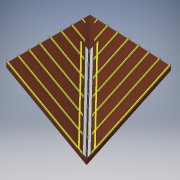
# Autodesk Inventor part: DeszkazatEsSzarufa
Saved by Autodesk Inventor 2019 (Build 230136000, 136)
## iProperties
Created: 2022-04-03
Part Number: DeszkazatEsSzarufa
Material: Generic
Document SubType Name: Modeling
Designer: laca
Density: 1 g/cm^3
Appearance: Default
Author: laca
Autodesk Inventor part; units mm, degrees
ref_plane "YZ Plane" through (0, 0, 0) normal (1, 0, 0) x (0, 1, 0)
ref_plane "XZ Plane" through (0, 0, 0) normal (0, 1, 0) x (-1, 0, 0)
ref_plane "XY Plane" through (0, 0, 0) normal (0, 0, 1) x (1, 0, 0)
sketch "Sketch1" plane through (0, 0, 0) normal (0, 0, 1) x (1, 0, 0)
  line L0 (0, 0) -> (-5247.7182, 2908.8577)
  line L1 (0, 0) -> (-5580.1481, 0)
  line L2 (0, 0) -> (-104.9544, 58.1772)
  line L3 (-104.9544, 58.1772) -> (-117.0746, 36.3117)
  line L4 (-117.0746, 36.3117) -> (-12.1202, -21.8655)
  line L5 (-12.1202, -21.8655) -> (0, 0)
  line L6 (-113.7006, 63.0253) -> (-218.6549, 121.2024)
  line L7 (-218.6549, 121.2024) -> (-230.7752, 99.3369)
  line L8 (-230.7752, 99.3369) -> (-125.8208, 41.1598)
  line L9 (-125.8208, 41.1598) -> (-113.7006, 63.0253)
  line L10 (-227.4011, 126.0505) -> (-332.3555, 184.2277)
  line L11 (-332.3555, 184.2277) -> (-344.4757, 162.3622)
  line L12 (-344.4757, 162.3622) -> (-239.5214, 104.185)
  line L13 (-239.5214, 104.185) -> (-227.4011, 126.0505)
  line L14 (-341.1017, 189.0758) -> (-446.0561, 247.2529)
  line L15 (-446.0561, 247.2529) -> (-458.1763, 225.3874)
  line L16 (-458.1763, 225.3874) -> (-353.2219, 167.2103)
  line L17 (-353.2219, 167.2103) -> (-341.1017, 189.0758)
  line L18 (-454.8022, 252.101) -> (-559.7566, 310.2782)
  line L19 (-559.7566, 310.2782) -> (-571.8769, 288.4127)
  line L20 (-571.8769, 288.4127) -> (-466.9225, 230.2355)
  line L21 (-466.9225, 230.2355) -> (-454.8022, 252.101)
  line L22 (-568.5028, 315.1263) -> (-673.4572, 373.3034)
  line L23 (-673.4572, 373.3034) -> (-685.5774, 351.4379)
  line L24 (-685.5774, 351.4379) -> (-580.6231, 293.2608)
  line L25 (-580.6231, 293.2608) -> (-568.5028, 315.1263)
  line L26 (-682.2034, 378.1515) -> (-787.1577, 436.3287)
  line L27 (-787.1577, 436.3287) -> (-799.278, 414.4632)
  line L28 (-799.278, 414.4632) -> (-694.3236, 356.286)
  line L29 (-694.3236, 356.286) -> (-682.2034, 378.1515)
  line L30 (-795.9039, 441.1768) -> (-900.8583, 499.3539)
  line L31 (-900.8583, 499.3539) -> (-912.9785, 477.4884)
  line L32 (-912.9785, 477.4884) -> (-808.0242, 419.3113)
  line L33 (-808.0242, 419.3113) -> (-795.9039, 441.1768)
  line L34 (-909.6045, 504.202) -> (-1014.5589, 562.3792)
  line L35 (-1014.5589, 562.3792) -> (-1026.6791, 540.5137)
  line L36 (-1026.6791, 540.5137) -> (-921.7247, 482.3365)
  line L37 (-921.7247, 482.3365) -> (-909.6045, 504.202)
  line L38 (-1023.3051, 567.2273) -> (-1128.2594, 625.4044)
  line L39 (-1128.2594, 625.4044) -> (-1140.3797, 603.5389)
  line L40 (-1140.3797, 603.5389) -> (-1035.4253, 545.3618)
  line L41 (-1035.4253, 545.3618) -> (-1023.3051, 567.2273)
  line L42 (-1137.0056, 630.2525) -> (-1241.96, 688.4297)
  line L43 (-1241.96, 688.4297) -> (-1254.0802, 666.5642)
  line L44 (-1254.0802, 666.5642) -> (-1149.1259, 608.387)
  line L45 (-1149.1259, 608.387) -> (-1137.0056, 630.2525)
  line L46 (-1250.7062, 693.2778) -> (-1355.6605, 751.4549)
  line L47 (-1355.6605, 751.4549) -> (-1367.7808, 729.5894)
  line L48 (-1367.7808, 729.5894) -> (-1262.8264, 671.4123)
  line L49 (-1262.8264, 671.4123) -> (-1250.7062, 693.2778)
  line L50 (-1364.4067, 756.303) -> (-1469.3611, 814.4802)
  line L51 (-1469.3611, 814.4802) -> (-1481.4813, 792.6147)
  line L52 (-1481.4813, 792.6147) -> (-1376.527, 734.4375)
  line L53 (-1376.527, 734.4375) -> (-1364.4067, 756.303)
  line L54 (-1478.1073, 819.3283) -> (-1583.0617, 877.5054)
  line L55 (-1583.0617, 877.5054) -> (-1595.1819, 855.6399)
  line L56 (-1595.1819, 855.6399) -> (-1490.2275, 797.4628)
  line L57 (-1490.2275, 797.4628) -> (-1478.1073, 819.3283)
  line L58 (-1591.8079, 882.3535) -> (-1696.7622, 940.5307)
  line L59 (-1696.7622, 940.5307) -> (-1708.8825, 918.6652)
  line L60 (-1708.8825, 918.6652) -> (-1603.9281, 860.488)
  line L61 (-1603.9281, 860.488) -> (-1591.8079, 882.3535)
  line L62 (-1705.5084, 945.3788) -> (-1810.4628, 1003.5559)
  line L63 (-1810.4628, 1003.5559) -> (-1822.583, 981.6904)
  line L64 (-1822.583, 981.6904) -> (-1717.6287, 923.5133)
  line L65 (-1717.6287, 923.5133) -> (-1705.5084, 945.3788)
  line L66 (-1819.209, 1008.404) -> (-1924.1634, 1066.5812)
  line L67 (-1924.1634, 1066.5812) -> (-1936.2836, 1044.7157)
  line L68 (-1936.2836, 1044.7157) -> (-1831.3292, 986.5385)
  line L69 (-1831.3292, 986.5385) -> (-1819.209, 1008.404)
  line L70 (-1932.9096, 1071.4293) -> (-2037.8639, 1129.6064)
  line L71 (-2037.8639, 1129.6064) -> (-2049.9842, 1107.7409)
  line L72 (-2049.9842, 1107.7409) -> (-1945.0298, 1049.5638)
  line L73 (-1945.0298, 1049.5638) -> (-1932.9096, 1071.4293)
  line L74 (-2046.6101, 1134.4545) -> (-2151.5645, 1192.6317)
  line L75 (-2151.5645, 1192.6317) -> (-2163.6847, 1170.7662)
  line L76 (-2163.6847, 1170.7662) -> (-2058.7304, 1112.589)
  line L77 (-2058.7304, 1112.589) -> (-2046.6101, 1134.4545)
  line L78 (-2160.3107, 1197.4798) -> (-2265.265, 1255.6569)
  line L79 (-2265.265, 1255.6569) -> (-2277.3853, 1233.7914)
  line L80 (-2277.3853, 1233.7914) -> (-2172.4309, 1175.6143)
  line L81 (-2172.4309, 1175.6143) -> (-2160.3107, 1197.4798)
  line L82 (-2274.0112, 1260.505) -> (-2378.9656, 1318.6822)
  line L83 (-2378.9656, 1318.6822) -> (-2391.0858, 1296.8167)
  line L84 (-2391.0858, 1296.8167) -> (-2286.1315, 1238.6395)
  line L85 (-2286.1315, 1238.6395) -> (-2274.0112, 1260.505)
  line L86 (-2387.7118, 1323.5303) -> (-2492.6662, 1381.7074)
  line L87 (-2492.6662, 1381.7074) -> (-2504.7864, 1359.8419)
  line L88 (-2504.7864, 1359.8419) -> (-2399.832, 1301.6648)
  line L89 (-2399.832, 1301.6648) -> (-2387.7118, 1323.5303)
  line L90 (-2501.4124, 1386.5555) -> (-2606.3667, 1444.7327)
  line L91 (-2606.3667, 1444.7327) -> (-2618.487, 1422.8672)
  line L92 (-2618.487, 1422.8672) -> (-2513.5326, 1364.69)
  line L93 (-2513.5326, 1364.69) -> (-2501.4124, 1386.5555)
  line L94 (-2615.1129, 1449.5808) -> (-2720.0673, 1507.7579)
  line L95 (-2720.0673, 1507.7579) -> (-2732.1875, 1485.8924)
  line L96 (-2732.1875, 1485.8924) -> (-2627.2332, 1427.7153)
  line L97 (-2627.2332, 1427.7153) -> (-2615.1129, 1449.5808)
  line L98 (-2728.8135, 1512.606) -> (-2833.7679, 1570.7832)
  line L99 (-2833.7679, 1570.7832) -> (-2845.8881, 1548.9177)
  line L100 (-2845.8881, 1548.9177) -> (-2740.9337, 1490.7405)
  line L101 (-2740.9337, 1490.7405) -> (-2728.8135, 1512.606)
  line L102 (-2842.514, 1575.6313) -> (-2947.4684, 1633.8084)
  line L103 (-2947.4684, 1633.8084) -> (-2959.5887, 1611.9429)
  line L104 (-2959.5887, 1611.9429) -> (-2854.6343, 1553.7658)
  line L105 (-2854.6343, 1553.7658) -> (-2842.514, 1575.6313)
  line L106 (-2956.2146, 1638.6565) -> (-3061.169, 1696.8337)
  line L107 (-3061.169, 1696.8337) -> (-3073.2892, 1674.9682)
  line L108 (-3073.2892, 1674.9682) -> (-2968.3349, 1616.791)
  line L109 (-2968.3349, 1616.791) -> (-2956.2146, 1638.6565)
  line L110 (-3069.9152, 1701.6818) -> (-3174.8695, 1759.8589)
  line L111 (-3174.8695, 1759.8589) -> (-3186.9898, 1737.9934)
  line L112 (-3186.9898, 1737.9934) -> (-3082.0354, 1679.8163)
  line L113 (-3082.0354, 1679.8163) -> (-3069.9152, 1701.6818)
  line L114 (-3183.6157, 1764.707) -> (-3288.5701, 1822.8842)
  line L115 (-3288.5701, 1822.8842) -> (-3300.6903, 1801.0187)
  line L116 (-3300.6903, 1801.0187) -> (-3195.736, 1742.8415)
  line L117 (-3195.736, 1742.8415) -> (-3183.6157, 1764.707)
  line L118 (-3297.3163, 1827.7323) -> (-3402.2707, 1885.9094)
  line L119 (-3402.2707, 1885.9094) -> (-3414.3909, 1864.0439)
  line L120 (-3414.3909, 1864.0439) -> (-3309.4365, 1805.8668)
  line L121 (-3309.4365, 1805.8668) -> (-3297.3163, 1827.7323)
  line L122 (-3411.0169, 1890.7575) -> (-3515.9712, 1948.9347)
  line L123 (-3515.9712, 1948.9347) -> (-3528.0915, 1927.0692)
  line L124 (-3528.0915, 1927.0692) -> (-3423.1371, 1868.892)
  line L125 (-3423.1371, 1868.892) -> (-3411.0169, 1890.7575)
  line L126 (-3524.7174, 1953.7828) -> (-3629.6718, 2011.9599)
  line L127 (-3629.6718, 2011.9599) -> (-3641.792, 1990.0944)
  line L128 (-3641.792, 1990.0944) -> (-3536.8377, 1931.9173)
  line L129 (-3536.8377, 1931.9173) -> (-3524.7174, 1953.7828)
  line L130 (-3638.418, 2016.808) -> (-3743.3723, 2074.9852)
  line L131 (-3743.3723, 2074.9852) -> (-3755.4926, 2053.1197)
  line L132 (-3755.4926, 2053.1197) -> (-3650.5382, 1994.9425)
  line L133 (-3650.5382, 1994.9425) -> (-3638.418, 2016.808)
  line L134 (-3752.1185, 2079.8333) -> (-3857.0729, 2138.0104)
  line L135 (-3857.0729, 2138.0104) -> (-3869.1931, 2116.1449)
  line L136 (-3869.1931, 2116.1449) -> (-3764.2388, 2057.9678)
  line L137 (-3764.2388, 2057.9678) -> (-3752.1185, 2079.8333)
  line L138 (-3865.8191, 2142.8585) -> (-3970.7735, 2201.0357)
  line L139 (-3970.7735, 2201.0357) -> (-3982.8937, 2179.1702)
  line L140 (-3982.8937, 2179.1702) -> (-3877.9393, 2120.993)
  line L141 (-3877.9393, 2120.993) -> (-3865.8191, 2142.8585)
  line L142 (-3979.5197, 2205.8838) -> (-4084.474, 2264.0609)
  line L143 (-4084.474, 2264.0609) -> (-4096.5943, 2242.1954)
  line L144 (-4096.5943, 2242.1954) -> (-3991.6399, 2184.0183)
  line L145 (-3991.6399, 2184.0183) -> (-3979.5197, 2205.8838)
  line L146 (-4093.2202, 2268.909) -> (-4198.1746, 2327.0862)
  line L147 (-4198.1746, 2327.0862) -> (-4210.2948, 2305.2207)
  line L148 (-4210.2948, 2305.2207) -> (-4105.3405, 2247.0435)
  line L149 (-4105.3405, 2247.0435) -> (-4093.2202, 2268.909)
  line L150 (-4206.9208, 2331.9343) -> (-4311.8752, 2390.1114)
  line L151 (-4311.8752, 2390.1114) -> (-4323.9954, 2368.2459)
  line L152 (-4323.9954, 2368.2459) -> (-4219.041, 2310.0688)
  line L153 (-4219.041, 2310.0688) -> (-4206.9208, 2331.9343)
  line L154 (-4320.6214, 2394.9595) -> (-4425.5757, 2453.1367)
  line L155 (-4425.5757, 2453.1367) -> (-4437.696, 2431.2712)
  line L156 (-4437.696, 2431.2712) -> (-4332.7416, 2373.094)
  line L157 (-4332.7416, 2373.094) -> (-4320.6214, 2394.9595)
  line L158 (-4434.3219, 2457.9848) -> (-4539.2763, 2516.1619)
  line L159 (-4539.2763, 2516.1619) -> (-4551.3965, 2494.2964)
  line L160 (-4551.3965, 2494.2964) -> (-4446.4422, 2436.1193)
  line L161 (-4446.4422, 2436.1193) -> (-4434.3219, 2457.9848)
  line L162 (-4548.0225, 2521.01) -> (-4652.9768, 2579.1872)
  line L163 (-4652.9768, 2579.1872) -> (-4665.0971, 2557.3217)
  line L164 (-4665.0971, 2557.3217) -> (-4560.1427, 2499.1445)
  line L165 (-4560.1427, 2499.1445) -> (-4548.0225, 2521.01)
  line L166 (-4661.723, 2584.0353) -> (-4766.6774, 2642.2124)
  line L167 (-4766.6774, 2642.2124) -> (-4778.7976, 2620.3469)
  line L168 (-4778.7976, 2620.3469) -> (-4673.8433, 2562.1698)
  line L169 (-4673.8433, 2562.1698) -> (-4661.723, 2584.0353)
  line L170 (-4775.4236, 2647.0605) -> (-4880.378, 2705.2377)
  line L171 (-4880.378, 2705.2377) -> (-4892.4982, 2683.3722)
  line L172 (-4892.4982, 2683.3722) -> (-4787.5438, 2625.195)
  line L173 (-4787.5438, 2625.195) -> (-4775.4236, 2647.0605)
  line L174 (-4889.1242, 2710.0858) -> (-4994.0785, 2768.2629)
  line L175 (-4994.0785, 2768.2629) -> (-5006.1988, 2746.3974)
  line L176 (-5006.1988, 2746.3974) -> (-4901.2444, 2688.2203)
  line L177 (-4901.2444, 2688.2203) -> (-4889.1242, 2710.0858)
  line L178 (-5002.8247, 2773.111) -> (-5107.7791, 2831.2882)
  line L179 (-5107.7791, 2831.2882) -> (-5119.8993, 2809.4227)
  line L180 (-5119.8993, 2809.4227) -> (-5014.945, 2751.2455)
  line L181 (-5014.945, 2751.2455) -> (-5002.8247, 2773.111)
  line L182 (-5116.5253, 2836.1363) -> (-5221.4797, 2894.3134)
  line L183 (-5221.4797, 2894.3134) -> (-5233.5999, 2872.4479)
  line L184 (-5233.5999, 2872.4479) -> (-5128.6455, 2814.2708)
  line L185 (-5128.6455, 2814.2708) -> (-5116.5253, 2836.1363)
  line L186 (-5233.5999, 2872.4479) -> (-5233.5999, 0)
  line L187 (-5233.5999, 0) -> (-4003.4926, 2219.1722)
  dimension "d0" = 6000
  dimension "d3" = 29
  dimension "d6" = 120
  dimension "d7" = 25
  dimension "d12" = 130
  constraints: 376 end point, 3 perpendicular, 3 point on line, 2 parallel, 1 horizontal, 361 other
  measures "d0" distance of L0.start L0.end
  measures "d3" angle of L1 L0
  measures "d6" distance of L3.end L4.end
  measures "d7" distance of L2.end L3.end
  measures "d12" distance of L2.end L6.end
sketch "Sketch2" plane through (0, 0, 0) normal (1, 0, 0) x (0, 1, 0)
  line L0 (0, 0) -> (2816.8294, -5297.6856)
  line L1 (0, 0) -> (0, -5725.5113)
  dimension "d1" = 6000
  dimension "d2" = 28
  constraints: 4 end point, 1 vertical
  measures "d1" distance of L0.start L0.end
  measures "d2" angle of L1 L0
ref_plane "Work Plane1" through (0, 0, 0) normal (-1, 0, 0) x (0, 0.4694716, -0.8829476)
ref_plane "Work Plane2" through (0, 0, 0) normal (0, 0, -1) x (-1, 0, 0)
ref_plane "Work Plane5" through (0, 0, 0) normal (-0.7183246, 0.0123391, 0.6955987) x (-0.6462958, 0.3582476, -0.6737658)
ref_plane "Work Plane3" through (0, 0, 0) normal (0, 0.8829476, 0.4694716) x (0, 0.4694716, -0.8829476)
ref_plane "Work Plane4" through (0, 0, 0) normal (-0.4848096, -0.8746197, 0) x (-0.8746197, 0.4848096, 0)
extrude "Extrusion1" add sketch "Sketch1" against normal up to surface contours L1 L4 L3 L0 | L5 L4 L1 | L9 L8 L7 L0 | L183 L0 L185 L184 | L187 L0 L145 L144 | L144 L143 L0 L187 | L13 L12 L11 L0 | L17 L16 L15 L0 | L0 L181 L180 L179 | L149 L148 L147 L0 | L0 L141 L140 L139 | L21 L20 L19 L0 | L0 L177 L176 L175 | L153 L152 L151 L0 | L0 L137 L136 L135 | L25 L24 L23 L0 | L0 L173 L172 L171 | L157 L156 L155 L0 | L0 L133 L132 L131 | L29 L28 L27 L0 | L0 L169 L168 L167 | L161 L160 L159 L0 | L0 L129 L128 L127 | L33 L32 L31 L0 | L0 L165 L164 L163 | L0 L125 L124 L123 | L37 L36 L35 L0 | L0 L121 L120 L119 | L41 L40 L39 L0 | L0 L117 L116 L115 | L45 L44 L43 L0 | L0 L113 L112 L111 | L49 L48 L47 L0 | L0 L109 L108 L107 | L53 L52 L51 L0 | L0 L105 L104 L103 | L57 L56 L55 L0 | L0 L101 L100 L99 | L61 L60 L59 L0 | L0 L97 L96 L95 | L65 L64 L63 L0 | L0 L93 L92 L91 | L69 L68 L67 L0 | L0 L89 L88 L87 | L73 L72 L71 L0 | L0 L85 L84 L83 | L77 L76 L75 L0 | L0 L81 L80 L79 surface through (0, 0, 0) normal (-0.7183246, 0.0123391, 0.6955987)
mirror "Mirror1" about plane through (0, 0, 0) normal (-0.7183246, 0.0123391, 0.6955987) of "Extrusion1"
ref_plane "Work Plane6" through (-5233.5999, 2872.4479, 0) normal (1, 0, 0) x (0, -1, 0)
ref_plane "Work Plane7" through (-5233.5999, 0, 0) normal (-0.8746197, 0.4848096, 0) x (0.4848096, 0.8746197, 0)
sketch "Sketch4" plane through (-5233.5999, 0, 0) normal (-0.8746197, 0.4848096, 0) x (0.4848096, 0.8746197, 0)
  line L0 (2512.2996, 0) -> (2512.2996, 595.6767) projected
  line L1 (2512.2996, 0) -> (2512.2996, 100)
  line L2 (2512.2996, 100) -> (2312.2996, 100)
  line L3 (2312.2996, 100) -> (2312.2996, 0)
  line L4 (2312.2996, 0) -> (2512.2996, 0)
  line L5 (2512.2996, 0) -> (2537.2996, 0) projected
  line L6 (2512.2996, 700) -> (2512.2996, 800)
  line L7 (2512.2996, 800) -> (2312.2996, 800)
  line L8 (2312.2996, 800) -> (2312.2996, 700)
  line L9 (2312.2996, 700) -> (2512.2996, 700)
  line L10 (2512.2996, 1400) -> (2512.2996, 1500)
  line L11 (2512.2996, 1500) -> (2312.2996, 1500)
  line L12 (2312.2996, 1500) -> (2312.2996, 1400)
  line L13 (2312.2996, 1400) -> (2512.2996, 1400)
  line L14 (2512.2996, 2100) -> (2512.2996, 2200)
  line L15 (2512.2996, 2200) -> (2312.2996, 2200)
  line L16 (2312.2996, 2200) -> (2312.2996, 2100)
  line L17 (2312.2996, 2100) -> (2512.2996, 2100)
  line L18 (2512.2996, 2800) -> (2512.2996, 2900)
  line L19 (2512.2996, 2900) -> (2312.2996, 2900)
  line L20 (2312.2996, 2900) -> (2312.2996, 2800)
  line L21 (2312.2996, 2800) -> (2512.2996, 2800)
  line L22 (2512.2996, 3500) -> (2512.2996, 3600)
  line L23 (2512.2996, 3600) -> (2312.2996, 3600)
  line L24 (2312.2996, 3600) -> (2312.2996, 3500)
  line L25 (2312.2996, 3500) -> (2512.2996, 3500)
  line L26 (2512.2996, 4200) -> (2512.2996, 4300)
  line L27 (2512.2996, 4300) -> (2312.2996, 4300)
  line L28 (2312.2996, 4300) -> (2312.2996, 4200)
  line L29 (2312.2996, 4200) -> (2512.2996, 4200)
  line L30 (2512.2996, 4900) -> (2512.2996, 5000)
  line L31 (2512.2996, 5000) -> (2312.2996, 5000)
  line L32 (2312.2996, 5000) -> (2312.2996, 4900)
  line L33 (2312.2996, 4900) -> (2512.2996, 4900)
  line L34 (2512.2996, 5600) -> (2512.2996, 5700)
  line L35 (2512.2996, 5700) -> (2312.2996, 5700)
  line L36 (2312.2996, 5700) -> (2312.2996, 5600)
  line L37 (2312.2996, 5600) -> (2512.2996, 5600)
  line L38 (2537.2996, 0) -> (2588.667, 105.8829) projected
  line L39 (2537.2996, 90) -> (2547.2996, 90)
  line L40 (2547.2996, 90) -> (2547.2996, 10)
  line L41 (2547.2996, 10) -> (2537.2996, 10)
  line L42 (2537.2996, 10) -> (2537.2996, 90)
  line L43 (2537.2996, 710) -> (2537.2996, 790)
  line L44 (2547.2996, 790) -> (2547.2996, 710)
  line L45 (2547.2996, 710) -> (2537.2996, 710)
  line L46 (2537.2996, 790) -> (2547.2996, 790)
  line L47 (2537.2996, 1410) -> (2537.2996, 1490)
  line L48 (2547.2996, 1490) -> (2547.2996, 1410)
  line L49 (2547.2996, 1410) -> (2537.2996, 1410)
  line L50 (2537.2996, 1490) -> (2547.2996, 1490)
  line L51 (2537.2996, 2110) -> (2537.2996, 2190)
  line L52 (2547.2996, 2190) -> (2547.2996, 2110)
  line L53 (2547.2996, 2110) -> (2537.2996, 2110)
  line L54 (2537.2996, 2190) -> (2547.2996, 2190)
  line L55 (2537.2996, 2810) -> (2537.2996, 2890)
  line L56 (2547.2996, 2890) -> (2547.2996, 2810)
  line L57 (2547.2996, 2810) -> (2537.2996, 2810)
  line L58 (2537.2996, 2890) -> (2547.2996, 2890)
  line L59 (2537.2996, 3510) -> (2537.2996, 3590)
  line L60 (2547.2996, 3590) -> (2547.2996, 3510)
  line L61 (2547.2996, 3510) -> (2537.2996, 3510)
  line L62 (2537.2996, 3590) -> (2547.2996, 3590)
  line L63 (2537.2996, 4210) -> (2537.2996, 4290)
  line L64 (2547.2996, 4290) -> (2547.2996, 4210)
  line L65 (2547.2996, 4210) -> (2537.2996, 4210)
  line L66 (2537.2996, 4290) -> (2547.2996, 4290)
  line L67 (2537.2996, 4910) -> (2537.2996, 4990)
  line L68 (2547.2996, 4990) -> (2547.2996, 4910)
  line L69 (2547.2996, 4910) -> (2537.2996, 4910)
  line L70 (2537.2996, 4990) -> (2547.2996, 4990)
  line L71 (2537.2996, 5610) -> (2537.2996, 5690)
  line L72 (2547.2996, 5690) -> (2547.2996, 5610)
  line L73 (2547.2996, 5610) -> (2537.2996, 5610)
  line L74 (2537.2996, 5690) -> (2547.2996, 5690)
  line L75 (2547.2996, 15) -> (2607.2996, 15)
  line L76 (2607.2996, 15) -> (2607.2996, 85)
  line L77 (2607.2996, 85) -> (2547.2996, 85)
  line L78 (2547.2996, 85) -> (2547.2996, 15)
  line L79 (2607.2996, 785) -> (2547.2996, 785)
  line L80 (2547.2996, 785) -> (2547.2996, 715)
  line L81 (2547.2996, 715) -> (2607.2996, 715)
  line L82 (2607.2996, 715) -> (2607.2996, 785)
  line L83 (2607.2996, 1485) -> (2547.2996, 1485)
  line L84 (2547.2996, 1485) -> (2547.2996, 1415)
  line L85 (2547.2996, 1415) -> (2607.2996, 1415)
  line L86 (2607.2996, 1415) -> (2607.2996, 1485)
  line L87 (2607.2996, 2185) -> (2547.2996, 2185)
  line L88 (2547.2996, 2185) -> (2547.2996, 2115)
  line L89 (2547.2996, 2115) -> (2607.2996, 2115)
  line L90 (2607.2996, 2115) -> (2607.2996, 2185)
  line L91 (2607.2996, 2885) -> (2547.2996, 2885)
  line L92 (2547.2996, 2885) -> (2547.2996, 2815)
  line L93 (2547.2996, 2815) -> (2607.2996, 2815)
  line L94 (2607.2996, 2815) -> (2607.2996, 2885)
  line L95 (2607.2996, 3585) -> (2547.2996, 3585)
  line L96 (2547.2996, 3585) -> (2547.2996, 3515)
  line L97 (2547.2996, 3515) -> (2607.2996, 3515)
  line L98 (2607.2996, 3515) -> (2607.2996, 3585)
  line L99 (2607.2996, 4285) -> (2547.2996, 4285)
  line L100 (2547.2996, 4285) -> (2547.2996, 4215)
  line L101 (2547.2996, 4215) -> (2607.2996, 4215)
  line L102 (2607.2996, 4215) -> (2607.2996, 4285)
  line L103 (2607.2996, 4985) -> (2547.2996, 4985)
  line L104 (2547.2996, 4985) -> (2547.2996, 4915)
  line L105 (2547.2996, 4915) -> (2607.2996, 4915)
  line L106 (2607.2996, 4915) -> (2607.2996, 4985)
  line L107 (2607.2996, 5685) -> (2547.2996, 5685)
  line L108 (2547.2996, 5685) -> (2547.2996, 5615)
  line L109 (2547.2996, 5615) -> (2607.2996, 5615)
  line L110 (2607.2996, 5615) -> (2607.2996, 5685)
  dimension "d18" = 200
  dimension "d19" = 100
  dimension "d20" = 0
  dimension "d23" = 700
  dimension "d33" = 80
  dimension "d34" = 10
  dimension "d35" = 10
  dimension "d36" = 25
  dimension "d41" = 700
  dimension "d67" = 70
  dimension "d68" = 60
  dimension "d69" = 5
  dimension "d72" = 700
  constraints: 216 end point, 6 parallel, 3 perpendicular, 3 vertical, 2 horizontal, 2 point on line, 1 collinear, 191 other
  measures "d18" distance of L1.end L2.end
  measures "d19" distance between parallel lines of L2 L4
  measures "d20" distance between parallel lines of L5 L4
  measures "d23" distance of L1.start L6.start
  measures "d33" distance of L39.end L40.end
  measures "d34" distance between parallel lines of L42 L40
  measures "d35" distance between parallel lines of L4 L41
  measures "d36" distance between parallel lines of L0 L42
  measures "d41" distance of L39.start L43.end
  measures "d67" distance of L75.end L76.end
  measures "d68" distance of L75.start L75.end
  measures "d69" distance between parallel lines of L75 L41
  measures "d72" distance of L77.end L79.end
extrude "Extrusion2" add sketch "Sketch4" against normal up to surface contours L4 L3 L2 L0 | L9 L8 L7 L6 | L13 L12 L11 L10 | L17 L16 L15 L14 | L21 L20 L19 L18 | L25 L24 L23 L22 | L29 L28 L27 L26 | L33 L32 L31 L30 starts on plane at (-5233.5999, 2872.4479, 0) facing (1, 0, 0) surface through (0, 0, 0) normal (-0.7183246, 0.0123391, 0.6955987)
mirror "Mirror2" about plane through (0, 0, 0) normal (-0.7183246, 0.0123391, 0.6955987) of "Extrusion2"
ref_plane "Work Plane14" through (-143.6649, 2.4678, 139.1197) normal (-0.7183246, 0.0123391, 0.6955987) x (-0.6462958, 0.3582476, -0.6737658)
extrude "Extrusion3" add sketch "Sketch4" along normal up to surface contours L29 L28 L27 L26 | L41 L42 L39 L40 L38 | L38 L40 L41 | L40 L77 L38 | L38 L77 L76 L75 L40 | L43 L46 L44 L45 | L44 L79 L82 L81 | L47 L50 L48 L49 | L48 L83 L86 L85 | L51 L54 L52 L53 | L52 L87 L90 L89 | L55 L58 L56 L57 | L56 L91 L94 L93 | L59 L62 L60 L61 | L60 L95 L98 L97 | L63 L66 L64 L65 | L64 L99 L102 L101 | L67 L70 L68 L69 starts on plane at (-143.6649, 2.4678, 139.1197) facing (-0.7183246, 0.0123391, 0.6955987) surface through (-5233.5999, 2872.4479, 0) normal (1, 0, 0)
mirror "Mirror3" about plane through (0, 0, 0) normal (-0.7183246, 0.0123391, 0.6955987) of "Extrusion3"
ref_plane "Work Plane8" through (26.6021, 1548.6459, 0) normal (-0.6954961, 0.011947, -0.7184305) x (-0.0171751, -0.9998525, 0)
ref_plane "Work Plane9" through (-4452.1422, 4282.235, -4673.5596) normal (0.5419856, -0.6169483, 0.5706368) x (0.4361896, 0.7869069, 0.4364815)
sketch "Sketch6" plane through (0, 0, 0) normal (-0.7183246, 0.0123391, 0.6955987) x (-0.6462958, 0.3582476, -0.6737658)
  line L0 (0, 0) -> (0, -2220.7686)
  constraints: 2 end point, 1 vertical
ref_plane "Work Plane12" through (0, 0, 0) normal (0.6462958, -0.3582476, 0.6737658) x (0.2575103, 0.9335451, 0.2493633)
sketch "Sketch7" plane through (0, 0, 0) normal (0.6462958, -0.3582476, 0.6737658) x (0.2575103, 0.9335451, 0.2493633)
  line L0 (670.5009, -1840.7282) -> (82.3206, -200) projected
  line L1 (24.119, -37.6466) -> (51.1157, -112.9539)
  line L2 (51.1157, -112.9539) -> (41.7023, -116.3285)
  line L3 (41.7023, -116.3285) -> (14.7056, -41.0212)
  line L4 (14.7056, -41.0212) -> (24.119, -37.6466)
  line L5 (825.1062, 2271.9994) -> (82.3206, 200) projected
  line L6 (91.6107, -225.9147) -> (118.6074, -301.2219)
  line L7 (118.6074, -301.2219) -> (109.194, -304.5965)
  line L8 (109.194, -304.5965) -> (82.1973, -229.2893)
  line L9 (82.1973, -229.2893) -> (91.6107, -225.9147)
  line L10 (25.8063, -42.3533) -> (49.4284, -108.2472)
  line L11 (49.4284, -108.2472) -> (105.9088, -87.9996)
  line L12 (105.9088, -87.9996) -> (82.2867, -22.1058)
  line L13 (82.2867, -22.1058) -> (25.8063, -42.3533)
  line L14 (1239.504, -3250.1621) -> (146.0595, -200) projected
  line L15 (92.4105, -50.346) -> (143.0293, -191.5471)
  line L16 (143.0293, -191.5471) -> (166.5628, -183.1106)
  line L17 (166.5628, -183.1106) -> (115.944, -41.9096)
  line L18 (115.944, -41.9096) -> (92.4105, -50.346)
  line L19 (733.2965, -1838.0967) -> (146.0595, -200) projected
  line L20 (190.2735, -323.3347) -> (224.0193, -417.4688)
  line L21 (224.0193, -417.4688) -> (200.4858, -425.9052)
  line L22 (200.4858, -425.9052) -> (166.74, -331.7712)
  line L23 (166.74, -331.7712) -> (190.2735, -323.3347)
  point P0 (0, 0)
  point P1 (10.6012, 0)
  point P2 (10.6012, 0)
  point P3 (78.0929, -188.2681)
  point P4 (82.3206, -200)
  point P5 (82.3206, 200)
  dimension "d53" = 80
  dimension "d54" = 10
  dimension "d55" = 40
  dimension "d61" = 200
  dimension "d77" = 60
  dimension "d78" = 70
  dimension "d79" = 5
  dimension "d100" = 25
  dimension "d104" = 150
  dimension "d105" = 0
  dimension "d106" = 100
  dimension "d108" = 25
  dimension "d125" = 110
  dimension "d127" = 250
  constraints: 40 end point, 9 parallel, 4 perpendicular, 4 point on line, 2 collinear, 1 coincident, 12 other
  measures "d53" distance of L2.end L3.end
  measures "d54" distance of L1.end L2.end
  measures "d55" distance from line of L4 point (10.601, 0)
  measures "d61" distance of L1.start L6.start
  measures "d77" distance of L12.end L10.start
  measures "d78" distance of L11.end L12.end
  measures "d79" distance between parallel lines of L4 L13
  measures "d100" distance between parallel lines of L15 L17
  measures "d104" distance of L16.end L17.end
  measures "d105" distance between parallel lines of L20 L15
  measures "d106" distance of L21.end L22.end
  measures "d108" distance between parallel lines of L22 L15
  measures "d125" distance between parallel lines of L16 L11
  measures "d127" distance between parallel lines of L11 L23
extrude "Extrusion4" add sketch "Sketch7" against normal blind 6000 contours L1 L2 L3 L4 | L13 L12 L11 L1 | L12 L18 L17 L16 L15 | L21 L22 L23 L14 starts on plane at (216.0982, 2761.6847, -5220.5992) facing (0.9993313, -0.0171662, 0.0322848)
mirror "Mirror4" about plane through (0, 0, 0) normal (-0.7183246, 0.0123391, 0.6955987) of "Extrusion4"
sketch "Sketch8" plane through (-4.3773, -254.8283, 0) normal (0.9993313, -0.0171662, 0.0322848) x (0.0322801, -0.0005545, -0.9994787)
  line L0 (565.0031, 555.4844) -> (459.065, 499.1184) projected
  line L1 (311.3673, 499.6651) -> (5284.8278, 3144.101) projected
  line L2 (428.2892, 561.8336) -> (490.0955, 594.6966)
  line L3 (490.0955, 594.6966) -> (476.0114, 621.185)
  line L4 (476.0114, 621.185) -> (414.205, 588.322)
  line L5 (414.205, 588.322) -> (428.2892, 561.8336)
  line L6 (754.9798, 735.538) -> (740.8956, 762.0265)
  line L7 (693.1735, 702.675) -> (754.9798, 735.538)
  line L8 (679.0893, 729.1635) -> (693.1735, 702.675)
  line L9 (740.8956, 762.0265) -> (679.0893, 729.1635)
  line L10 (1019.8641, 876.3795) -> (1005.7799, 902.8679)
  line L11 (958.0577, 843.5165) -> (1019.8641, 876.3795)
  line L12 (943.9736, 870.0049) -> (958.0577, 843.5165)
  line L13 (1005.7799, 902.8679) -> (943.9736, 870.0049)
  line L14 (1284.7483, 1017.221) -> (1270.6642, 1043.7094)
  line L15 (1222.942, 984.358) -> (1284.7483, 1017.221)
  line L16 (1208.8579, 1010.8464) -> (1222.942, 984.358)
  line L17 (1270.6642, 1043.7094) -> (1208.8579, 1010.8464)
  line L18 (1549.6326, 1158.0624) -> (1535.5485, 1184.5509)
  line L19 (1487.8263, 1125.1994) -> (1549.6326, 1158.0624)
  line L20 (1473.7421, 1151.6879) -> (1487.8263, 1125.1994)
  line L21 (1535.5485, 1184.5509) -> (1473.7421, 1151.6879)
  line L22 (1814.5169, 1298.9039) -> (1800.4328, 1325.3923)
  line L23 (1752.7106, 1266.0409) -> (1814.5169, 1298.9039)
  line L24 (1738.6264, 1292.5293) -> (1752.7106, 1266.0409)
  line L25 (1800.4328, 1325.3923) -> (1738.6264, 1292.5293)
  line L26 (2079.4012, 1439.7454) -> (2065.317, 1466.2338)
  line L27 (2017.5948, 1406.8824) -> (2079.4012, 1439.7454)
  line L28 (2003.5107, 1433.3708) -> (2017.5948, 1406.8824)
  line L29 (2065.317, 1466.2338) -> (2003.5107, 1433.3708)
  line L30 (2344.2855, 1580.5869) -> (2330.2013, 1607.0753)
  line L31 (2282.4791, 1547.7238) -> (2344.2855, 1580.5869)
  line L32 (2268.395, 1574.2123) -> (2282.4791, 1547.7238)
  line L33 (2330.2013, 1607.0753) -> (2268.395, 1574.2123)
  line L34 (2609.1697, 1721.4283) -> (2595.0856, 1747.9167)
  line L35 (2547.3634, 1688.5653) -> (2609.1697, 1721.4283)
  line L36 (2533.2793, 1715.0537) -> (2547.3634, 1688.5653)
  line L37 (2595.0856, 1747.9167) -> (2533.2793, 1715.0537)
  line L38 (2874.054, 1862.2698) -> (2859.9699, 1888.7582)
  line L39 (2812.2477, 1829.4068) -> (2874.054, 1862.2698)
  line L40 (2798.1635, 1855.8952) -> (2812.2477, 1829.4068)
  line L41 (2859.9699, 1888.7582) -> (2798.1635, 1855.8952)
  line L42 (3138.9383, 2003.1113) -> (3124.8541, 2029.5997)
  line L43 (3077.132, 1970.2482) -> (3138.9383, 2003.1113)
  line L44 (3063.0478, 1996.7367) -> (3077.132, 1970.2482)
  line L45 (3124.8541, 2029.5997) -> (3063.0478, 1996.7367)
  line L46 (3403.8226, 2143.9527) -> (3389.7384, 2170.4412)
  line L47 (3342.0162, 2111.0897) -> (3403.8226, 2143.9527)
  line L48 (3327.9321, 2137.5781) -> (3342.0162, 2111.0897)
  line L49 (3389.7384, 2170.4412) -> (3327.9321, 2137.5781)
  line L50 (3668.7068, 2284.7942) -> (3654.6227, 2311.2826)
  line L51 (3606.9005, 2251.9312) -> (3668.7068, 2284.7942)
  line L52 (3592.8164, 2278.4196) -> (3606.9005, 2251.9312)
  line L53 (3654.6227, 2311.2826) -> (3592.8164, 2278.4196)
  line L54 (3933.5911, 2425.6357) -> (3919.507, 2452.1241)
  line L55 (3871.7848, 2392.7727) -> (3933.5911, 2425.6357)
  line L56 (3857.7006, 2419.2611) -> (3871.7848, 2392.7727)
  line L57 (3919.507, 2452.1241) -> (3857.7006, 2419.2611)
  line L58 (4198.4754, 2566.4771) -> (4184.3913, 2592.9656)
  line L59 (4136.6691, 2533.6141) -> (4198.4754, 2566.4771)
  line L60 (4122.5849, 2560.1026) -> (4136.6691, 2533.6141)
  line L61 (4184.3913, 2592.9656) -> (4122.5849, 2560.1026)
  line L62 (4463.3597, 2707.3186) -> (4449.2755, 2733.807)
  line L63 (4401.5533, 2674.4556) -> (4463.3597, 2707.3186)
  line L64 (4387.4692, 2700.944) -> (4401.5533, 2674.4556)
  line L65 (4449.2755, 2733.807) -> (4387.4692, 2700.944)
  line L66 (4728.244, 2848.1601) -> (4714.1598, 2874.6485)
  line L67 (4666.4376, 2815.2971) -> (4728.244, 2848.1601)
  line L68 (4652.3535, 2841.7855) -> (4666.4376, 2815.2971)
  line L69 (4714.1598, 2874.6485) -> (4652.3535, 2841.7855)
  line L70 (4993.1282, 2989.0015) -> (4979.0441, 3015.49)
  line L71 (4931.3219, 2956.1385) -> (4993.1282, 2989.0015)
  line L72 (4917.2378, 2982.627) -> (4931.3219, 2956.1385)
  line L73 (4979.0441, 3015.49) -> (4917.2378, 2982.627)
  line L74 (5258.0125, 3129.843) -> (5243.9284, 3156.3314)
  line L75 (5196.2062, 3096.98) -> (5258.0125, 3129.843)
  line L76 (5182.122, 3123.4684) -> (5196.2062, 3096.98)
  line L77 (5243.9284, 3156.3314) -> (5182.122, 3123.4684)
  line L78 (5522.8968, 3270.6845) -> (5508.8126, 3297.1729)
  line L79 (5461.0905, 3237.8215) -> (5522.8968, 3270.6845)
  line L80 (5447.0063, 3264.3099) -> (5461.0905, 3237.8215)
  line L81 (5508.8126, 3297.1729) -> (5447.0063, 3264.3099)
  point P0 (0, 254.8659)
  point P1 (5284.0281, 3145.6051)
  point P2 (292.9079, 490.0036)
  dimension "d88" = 30
  dimension "d89" = 70
  dimension "d90" = 522.2695
  dimension "d95" = 300
  constraints: 160 end point, 2 parallel, 1 collinear, 1 perpendicular, 154 other
  measures "d88" distance of L2.end L3.end
  measures "d89" distance of L3.end L4.end
  measures "d90" distance from line of point (0, 254.866) L5
  measures "d95" distance of L2.end L6.start
extrude "Extrusion5" [suppressed]
mirror "Mirror5" [suppressed]
sketch "Sketch9" plane through (214.2385, 2550.1961, -5275.4836) normal (0.9993313, -0.0171662, 0.0322848) x (0.0319803, -0.017727, -0.9993313)
  line L0 (-5229.2225, -2898.6054) -> (-5447.8384, -93.581) projected
  line L1 (-5242.4318, -2729.1194) -> (-5266.4318, -2729.1194)
  line L2 (-5276.6244, -2719.3157) -> (-5276.6244, -2559.1194)
  line L3 (-5276.6244, -2559.1194) -> (-5242.4318, -2559.1194)
  line L4 (-5242.4318, -2559.1194) -> (-5242.4318, -2729.1194)
  arc A0 (-5266.4318, -2729.1194) -> (-5276.6244, -2719.3157) centre (-5276.4299, -2729.3138) ccw
  point P0 (-5233.5999, -2643.7771)
  point P1 (-5447.8384, -93.581)
  dimension "d111" = 170
  dimension "d112" = 24
  dimension "d113" = 170
  dimension "d114" = 20
  constraints: 8 end point, 2 parallel, 2 point on circle, 1 centre point, 1 horizontal, 1 perpendicular, 2 other
  measures "d111" distance between parallel lines of L1 L3
  measures "d112" distance of L1.start L1.end
  measures "d113" distance of point (-5229.223, -2898.605) L1.start
  measures "d114" diameter of A0
sketch3d "3D Sketch1"
sweep "Sweep1" [suppressed]
sketch "Sketch10" plane through (0, 0, 0) normal (0, 0, 1) x (1, 0, 0)
  line L0 (-849.8479, 213.8237) -> (-500, 19.8999)
  line L1 (-4.3773, -254.8283) -> (-100.3003, -201.6573) projected
  line L2 (0, -86.1365) -> (0, -76.1602) projected
  point P0 (0, 0)
  point P1 (-9.3058, -86.1365)
  point P2 (-9.7491, -76.1602)
  dimension "d117" = 400
  dimension "d118" = 500
  constraints: 2 end point, 1 point on line
  measures "d117" distance of L0.start L0.end
  measures "d118" distance from line of L2 L0.end
sketch "Sketch11" plane through (-9.7491, -76.1602, 63.0645) normal (0.0289874, 0.0482431, 0.9984149) x (0.9980872, -0.0559602, -0.0262739)
  line L0 (55.4894, 130.1491) -> (55.4894, -29.2914)
  line L1 (0, 0) -> (-5279.69, 2787.0148) projected
  line L2 (-360.4673, 186.3315) -> (-360.4673, 345.772)
  line L3 (-311.3673, 319.6651) -> (-428.2892, 381.8336) projected
  line L4 (-360.4673, 186.3315) -> (55.4894, -29.2914)
  line L5 (-360.4673, 345.772) -> (55.4894, 130.1491)
  point P0 (7.1255, 79.6233)
  constraints: 8 end point, 2 parallel, 2 point on line, 1 vertical
extrude "Extrusion7" [suppressed]
equation "\"d35\" = -0.5 * d33 + 0.5 * d19"
equation "\"d69\" = -0.5 * d67 + 0.5 * d33"
equation "\"d79\" = -0.5 * d78 + 0.5 * d53"
body "Solid1"
